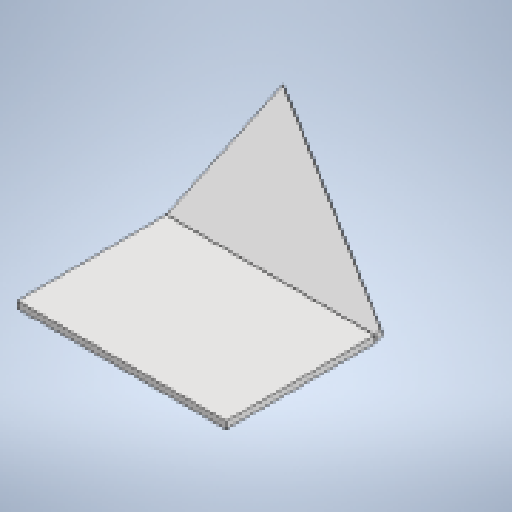
# Autodesk Inventor part: NVPH-307 left side
Saved by Autodesk Inventor 2025.1 (Build 291241020, 241B)
## iProperties
Created: 2024-12-03
Part Number: NVPH-307 left side
Material: Generic
Document SubType Name: Sheet Metal
Designer: user
Mass: 1002.11 g
Surface Area: 2135.82 cm^2
Volume: 1002.11 cm^3
Density: 1 g/cm^3
Flat Pattern Width: 31 cm
Flat Pattern Length: 41.4 cm
Flat Pattern Area: 1283.4 cm^2
Sheet Metal Rule: Default
Sheet Metal Width: 310.000 mm
Sheet Metal Length: 414.000 mm
Sheet Metal Area: 128340.000 mm^2
Appearance: Default
Author: user
Autodesk Inventor part; units mm, degrees
ref_plane "YZ Plane" through (0, 0, 0) normal (1, 0, 0) x (0, 1, 0)
ref_plane "XZ Plane" through (0, 0, 0) normal (0, 1, 0) x (-1, 0, 0)
ref_plane "XY Plane" through (0, 0, 0) normal (0, 0, 1) x (1, 0, 0)
sketch "Sketch3" plane through (0, 0, 0) normal (0, 0, 1) x (1, 0, 0)
  line L0 (0, 0) -> (-310, 0)
  line L1 (-310, 0) -> (-310, 232)
  line L2 (-310, 232) -> (0, 232)
  line L3 (0, 232) -> (0, 0)
  line L4 (0, 232) -> (-310, 414)
  line L5 (-310, 414) -> (-310, 232)
  dimension "d19" = 310
  dimension "d29" = 232
  dimension "d30" = 182
  measures "d19" distance of L0.start L0.end
  measures "d29" distance between parallel lines of L0 L2
  measures "d30" distance of L1.end L4.end
extrude "Plate3" add sketch "Sketch3" along normal blind 10
sketch "Sketch4" plane through (0, 0, 0) normal (0, 0, -1) x (-1, 0, 0)
  line L0 (310, 414) -> (310, 0) construction
  line L1 (0, 232) -> (310, 414) construction
  line L2 (0, 0) -> (0, 232) construction
  line L3 (310, 0) -> (0, 0) construction
  line L4 (0, 222) -> (310, 222)
  dimension "d22" = 10
  constraints: 2 end point, 2 point on line, 1 perpendicular
  measures "d22" distance from line of L4 L1.start
fold "Fold1" angle 25 bend radius 1 thickness 10 k factor 0.44 line from (0, 222, 0) to (-310, 222, 0) line at bend centre moving side (0, 1, 0) folds toward (0, 0, 1)
equation "\"d18\" = Thickness"
equation "\"d23\" = BendReliefWidth"
equation "\"d24\" = BendReliefDepth"
equation "\"d25\" = MinimumRemnant"
equation "\"d26\" = TransitionRadius"
equation "\"BendReliefDepth\" = 0.5 * Thickness"
equation "\"Thickness\" = 10"
equation "\"BendReliefWidth\" = 10"
equation "\"MinimumRemnant\" = 20"
equation "\"TransitionRadius\" = 10"
body "Solid2"
